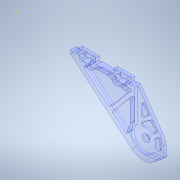
# Autodesk Inventor part: 後ろウィング固定フレームver2
Saved by Autodesk Inventor 2020.2 (Build 242310000, 310)
## iProperties
Created: 2020-05-07
Part Number: 後ろウィング固定フレームver2
Material: ポリカーボネート、クリア
Document SubType Name: Modeling
Designer: mozar
Density: 1.2 g/cm^3
Appearance: ポリカーボネート - クリア
Mass: 7.61117 g
Surface Area: 65.4566 cm^2
Volume: 6.34264 cm^3
Author: mozar
Autodesk Inventor part; units mm, degrees
(part 1 of 2)
ref_plane "YZ Plane" through (0, 0, 0) normal (1, 0, 0) x (0, 1, 0)
ref_plane "XZ Plane" through (0, 0, 0) normal (0, 1, 0) x (-1, 0, 0)
ref_plane "XY Plane" through (0, 0, 0) normal (0, 0, 1) x (1, 0, 0)
sketch "スケッチ1" plane through (0, 0, 0) normal (0, 0, 1) x (1, 0, 0)
  line L0 (-101.5, 48) -> (108.5, 48)
  circle A0 centre (111.885, -39) radius 4
  circle A1 centre (191.8767, -37.843) radius 4
  circle A2 centre (111.885, -39) radius 7
  circle A3 centre (191.8767, -37.843) radius 7
  line L1 (191.8767, -37.843) -> (111.885, -39) construction
  line L2 (191.7754, -30.8437) -> (111.7838, -32.0007)
  line L3 (111.9863, -45.9993) -> (191.9779, -44.8422)
  arc A4 (191.9779, -44.8422) -> (191.7754, -30.8437) centre (191.8767, -37.843) ccw
  arc A5 (111.7838, -32.0007) -> (111.9863, -45.9993) centre (111.885, -39) ccw
  line L4 (193.5423, -31.044) -> (241.7048, -42.843)
  circle A6 centre (234.5664, -71.9813) radius 30
  line L5 (262.5874, -82.6971) -> (213.7253, -50.4025)
  line L6 (213.7253, -50.4025) -> (190.2111, -44.6419)
  line L7 (264.5664, -121.5429) -> (264.5664, -63.2267)
  line L8 (111.885, -39) -> (111.885, 41) construction
  line L9 (118.885, -39) -> (118.885, 41)
  line L10 (104.885, 41) -> (104.885, -39)
  arc A7 (104.885, -39) -> (118.885, -39) centre (111.885, -39) ccw
  arc A8 (118.885, 41) -> (104.885, 41) centre (111.885, 41) ccw
  circle A9 centre (58.2383, 51.482) radius 30
  line L11 (113.5581, 34.2029) -> (65.4084, 22.3514)
  line L12 (28.4411, 48) -> (86.7041, 42.0109)
  line L13 (86.7041, 42.0109) -> (110.212, 47.7971)
  circle A10 centre (113.5, -20) radius 68
  line L14 (315.3272, -100.5855) -> (70.6004, 104.7647)
  line L15 (253.8501, -49) -> (111.885, -39)
  arc A11 (93.5924, -27.1048) -> (135.371, -5.9244) centre (95.0604, 21.7941) ccw
  arc A12 (135.371, -5.9244) -> (135.8476, -3.6716) centre (132.899, -4.2246) ccw
  arc A13 (135.8476, -3.6716) -> (83.1833, 18.5565) centre (102.1579, -9.9896) ccw
  line L16 (111.885, -39) -> (112.7472, 40.9954) construction
  line L17 (118.8846, -39.0754) -> (119.7468, 40.9199)
  line L18 (105.7476, 41.0708) -> (104.8855, -38.9246)
  arc A14 (104.8855, -38.9246) -> (118.8846, -39.0754) centre (111.885, -39) ccw
  arc A15 (119.7468, 40.9199) -> (105.7476, 41.0708) centre (112.7472, 40.9954) ccw
  line L19 (164.9949, 48) -> (164.9949, 26)
  line L20 (164.9949, 26) -> (327.4949, -102)
  circle A16 centre (116.2926, -40) radius 68
  circle A17 centre (-98.885, 0) radius 67.5
  line L21 (321.3633, -8.501) -> (-152.6681, 78.4982)
  line L22 (104.8897, -3) -> (104.8897, 0)
  line L23 (104.8897, -3) -> (64.4443, -3)
  line L24 (72.0656, 0) -> (104.8897, 0)
  circle A18 centre (83.3769, -17.5) radius 13.85
  line L25 (198.5102, -35.6076) -> (190.7791, -12.6656)
  line L26 (185.2432, -40.0784) -> (169.4082, 6.912)
  circle A19 centre (197.8374, 16.4922) radius 30
  line L27 (190.7791, -12.6656) -> (191.8767, 45.8941)
  circle A20 centre (191.8767, -37.843) radius 83.7371
  line L28 (191.8767, 45.8941) -> (191.8767, -37.843)
  line L29 (96.8897, -3) -> (96.8897, -6)
  line L30 (96.8897, -6) -> (87.8897, -6)
  line L31 (87.8897, -6) -> (87.8897, -3)
  line L32 (76.4443, -3) -> (76.4443, -6)
  line L33 (76.4443, -6) -> (67.4443, -6)
  line L34 (67.4443, -6) -> (67.4443, -3)
  line L35 (99.8897, -3) -> (99.8897, 0)
  line L36 (99.8897, 0) -> (84.8897, 0)
  line L37 (84.8897, 0) -> (84.8897, -3)
  line L38 (79.4443, -3) -> (79.4443, 0)
  line L39 (79.4443, 0) -> (64.4443, 0)
  line L40 (64.4443, 0) -> (64.4443, -3)
  line L41 (64.4443, 0) -> (59.4443, 0)
  line L42 (59.4443, 0) -> (59.4443, -3)
  line L43 (59.4443, -3) -> (64.4443, -3)
  line L44 (59.4443, -3) -> (59.4443, -6)
  circle A21 centre (111.885, -39) radius 1.5
  circle A22 centre (111.885, -39) radius 9
  circle A23 centre (111.885, -39) radius 10
  circle A24 centre (111.885, -39) radius 15
  line L45 (121.0577, -50.8686) -> (142.9273, -50.5523)
  line L46 (121.0577, -50.8686) -> (127.6513, -45.7727)
  line L47 (127.6513, -45.7727) -> (126.8081, -37.4821)
  line L48 (124.1514, -30.3665) -> (104.8897, -3)
  line L49 (101.0602, -49.3838) -> (59.4443, -6)
  circle A25 centre (95.8897, -6) radius 1
  circle A26 centre (88.8897, -6) radius 1
  circle A27 centre (95.8897, -3) radius 1
  circle A28 centre (88.8897, -3) radius 1
  circle A29 centre (100.8897, -3) radius 1
  circle A30 centre (83.8897, -3) radius 1
  circle A31 centre (80.4443, -3) radius 1
  circle A32 centre (75.4443, -6) radius 1
  circle A33 centre (68.4443, -6) radius 1
  circle A34 centre (75.4443, -3) radius 1
  circle A35 centre (68.4443, -3) radius 1
  circle A36 centre (63.4443, -3) radius 1
  point P0 (0, 0)
  point P1 (151.8809, -38.4215)
  point P2 (111.885, 1)
  point P3 (105.885, 0)
  point P4 (105.885, 0)
  point P5 (23.7328, -42.729)
  point P6 (112.3161, 0.9977)
  point P7 (99.8897, -1.5)
  point P8 (76.4443, -4.5)
  point P9 (74.4443, -6)
  point P10 (69.4443, -6)
  point P11 (69.4443, -3)
  point P12 (74.4443, -3)
  point P13 (82.8897, -3)
  point P14 (81.4443, -3)
  point P15 (62.4443, -3)
  point P16 (101.8897, -3)
  point P17 (89.8897, -3)
  point P18 (94.8897, -3)
  point P19 (94.8897, -6)
  point P20 (89.8897, -6)
  point P21 (118.9616, -31.9344)
  point P22 (118.9245, -31.8974)
  point P23 (118.962, -31.8969)
  point P24 (119.127, -45.896)
  point P25 (104.885, -3)
  point P26 (104.885, -31.8586)
  dimension "d27" = 167.4741
  dimension "d0" = 8
  dimension "d1" = 8
  dimension "d2" = 3
  dimension "d3" = 3
  dimension "d4" = 80
  dimension "d5" = 14
  dimension "d6" = 14
  dimension "d7" = 60
  dimension "d8" = 14
  dimension "d9" = 60
  dimension "d10" = 14
  dimension "d11" = 6
  dimension "d12" = 40
  dimension "d13" = 13.271
  dimension "d14" = 14
  dimension "d15" = 10
  dimension "d16" = 5
  dimension "d17" = 22
  dimension "d18" = 150
  dimension "d19" = 162.5
  dimension "d20" = 0
  dimension "d21" = 136
  dimension "d22" = 136
  dimension "d23" = 135
  dimension "d24" = 38.227
  dimension "d25" = 25
  dimension "d26" = 60
  dimension "d28" = 5
  dimension "d29" = 3
  dimension "d30" = 5
  dimension "d31" = 3
  dimension "d32" = 3
  dimension "d33" = 5
  dimension "d34" = 1
  dimension "d35" = 5
  dimension "d36" = 5
  dimension "d37" = 2
  dimension "d38" = 2
  dimension "d39" = 2
  dimension "d40" = 2
  dimension "d41" = 2
  dimension "d42" = 2
  dimension "d43" = 2
  dimension "d44" = 2
  dimension "d45" = 2
  dimension "d46" = 2
  dimension "d47" = 2
  dimension "d48" = 2
  constraints: 104 end point, 46 tangent, 37 point on circle, 36 centre point, 14 vertical, 8 point on line, 7 equal length, 7 horizontal, 5 coincident, 5 midpoint, 5 parallel, 1 concentric, 1 perpendicular, 1 vertical alignment, 25 other
  measures "d0" diameter of A0
  measures "d1" diameter of A1
  measures "d2" radial gap between concentric circles of A0 A2
  measures "d3" radial gap between concentric circles of A1 A3
  measures "d4" distance of L1.start L1.end
  measures "d5" diameter of A5
  measures "d6" distance from line of L4 L5.end
  measures "d7" diameter of A6
  measures "d8" diameter of A8
  measures "d9" diameter of A9
  measures "d10" distance from line of L11 L12.end
  measures "d11" horizontal distance of L1.end point (105.885, 0)
  measures "d12" angle of L14 L0
  measures "d14" diameter of A15
  measures "d15" vertical distance of L15.start L1.end
  measures "d16" vertical distance of L1.start L4.end
  measures "d17" distance of L19.start L19.end
  measures "d18" vertical distance of L19.start L20.end
  measures "d19" distance from line of L19 L20.end
  measures "d20" distance from line of L19.start L0
  measures "d21" diameter of A10
  measures "d22" diameter of A16
  measures "d23" diameter of A17
  measures "d24" angle of L0 L20
  measures "d25" distance from line of L5.start L20
  measures "d26" diameter of A19
  measures "d28" distance between parallel lines of L35 L22
  measures "d29" distance of L41.end L42.end
  measures "d30" distance of L42.end L40.end
  measures "d31" distance of L42.end L44.end
  measures "d32" diameter of A21
  measures "d33" radial gap between concentric circles of A0 A22
  measures "d34" radial gap between concentric circles of A22 A23
  measures "d35" radial gap between concentric circles of A23 A24
  measures "d36" distance between parallel lines of L3 L45
  measures "d37" diameter of A25
  measures "d38" diameter of A26
  measures "d39" diameter of A27
  measures "d40" diameter of A28
  measures "d41" diameter of A29
  measures "d42" diameter of A30
  measures "d43" diameter of A31
  measures "d44" diameter of A32
  measures "d45" diameter of A33
  measures "d46" diameter of A34
  measures "d47" diameter of A35
  measures "d48" diameter of A36
extrude "押し出し1" add sketch "スケッチ1" against normal blind 5 contours A24 A11 L10 A23 A20 | A20 A23 L3 A24 | L43 A36 L23 L34 A33 L33 A32 A18 L49 L44 | L46 A24 L3 | L3 A24 L15 L47 | A23 L10 A22 A20 | A20 A22 L3 A23 | L49 A18 L30 A25 L29 L23 A29 L10 A24 | L39 L24 L38 L23 A34 A35 L40 | L3 A23 L15 A24 | L15 A24 L47 | A22 L10 A2 A20 | A20 A2 L3 A22 | A23 L18 A22 L10 | L10 A11 L18 A23 | L3 A22 L15 A23 | A24 L10 A11 | L49 A18 A32 L32 A31 A30 L31 A26 L30 | L15 A23 L17 L2 A24 | L2 L17 A24 | A20 A0 L15 A2 | A2 A20 A0 | A22 L18 L10 | L3 A2 L15 A22 | L10 A24 L18 A11 | A23 A20 A22 L18 | L18 A11 A20 A23 | L15 A22 L17 A23 | L10 L23 L48 L18 A24 | L35 L23 A27 A28 L37 L24 | L48 A20 A24 L18 | L17 A23 L2 | L2 A23 L9 A24 L17 | A24 L17 L48 | A20 A0 | A0 A20 | L18 A22 A20 A2 | L15 A2 L17 A22 | L18 A24 A20 A11 | A23 L9 L2 A22 A20 | A20 A11 A24 L9 A23 | A31 A18 L32 L23 | L48 A11 A24 A20 | A23 L17 A22 L9 L2 | L2 L9 A23 | A24 L9 L48 L17 | L15 A0 A20 A2 | A20 A22 L2 A2 | A20 A24 A11 | A18 A30 L23 L31 | L23 A30 A18 A31 | L48 L9 A24 A11 | L9 A22 L2 | L17 L9 A22 | L2 A22 L9 A2
extrude "押し出し2" cut sketch "スケッチ1" against normal blind 2.55 contours L3 A24 L15 L47 | A23 L10 A22 A20 | A20 A22 L3 A23 | L3 A23 L15 A24 | L15 A24 L47 | A22 L10 A2 A20 | A20 A2 L3 A22 | A23 L18 A22 L10 | L10 A11 L18 A23 | L3 A22 L15 A23 | L15 A23 L17 L2 A24 | L2 L17 A24 | A20 A0 L15 A2 | A2 A20 A0 | A22 L18 L10 | L3 A2 L15 A22 | L10 A24 L18 A11 | A23 A20 A22 L18 | L18 A11 A20 A23 | L15 A22 L17 A23 | L10 L23 L48 L18 A24 | L48 A20 A24 L18 | L17 A23 L2 | L2 A23 L9 A24 L17 | A24 L17 L48 | A20 A0 | A0 A20 | L18 A22 A20 A2 | L15 A2 L17 A22 | L18 A24 A20 A11 | A23 L9 L2 A22 A20 | A20 A11 A24 L9 A23 | L48 A11 A24 A20 | A23 L17 A22 L9 L2 | L2 L9 A23 | A24 L9 L48 L17 | L15 A0 A20 A2 | A20 A22 L2 A2 | A20 A24 A11 | L48 L9 A24 A11 | L9 A22 L2 | L17 L9 A22 | L2 A22 L9 A2 | A21
sketch "スケッチ2" plane through (0, 0, 0) normal (0, 0, 1) x (1, 0, 0)
  line L0 (87.8897, -6) -> (87.8897, -3) projected
  arc A0 (89.8897, -3) -> (87.8897, -3) centre (88.8897, -3) ccw projected
  line L1 (89.8897, -3) -> (94.8897, -3) projected
  arc A1 (96.8897, -3) -> (94.8897, -3) centre (95.8897, -3) ccw projected
  line L2 (96.8897, -3) -> (96.8897, -6) projected
  arc A2 (94.8897, -6) -> (96.8897, -6) centre (95.8897, -6) ccw projected
  line L3 (94.8897, -6) -> (89.8897, -6) projected
  arc A3 (87.8897, -6) -> (89.8897, -6) centre (88.8897, -6) ccw projected
  arc A4 (67.4443, -6) -> (69.4443, -6) centre (68.4443, -6) ccw projected
  line L4 (67.4443, -6) -> (67.4443, -3) projected
  arc A5 (69.4443, -3) -> (67.4443, -3) centre (68.4443, -3) ccw projected
  line L5 (69.4443, -3) -> (74.4443, -3) projected
  arc A6 (76.4443, -3) -> (74.4443, -3) centre (75.4443, -3) ccw projected
  line L6 (76.4443, -3) -> (76.4443, -6) projected
  arc A7 (74.4443, -6) -> (76.4443, -6) centre (75.4443, -6) ccw projected
  line L7 (74.4443, -6) -> (69.4443, -6) projected
  line L8 (127.6513, -45.7727) -> (119.127, -45.896) projected
  arc A8 (104.885, -31.8586) -> (119.127, -45.896) centre (111.885, -39) ccw projected
  line L9 (104.885, -31.8586) -> (104.885, -3) projected
  line L10 (104.885, -3) -> (101.8897, -3) projected
  arc A9 (99.8897, -3) -> (101.8897, -3) centre (100.8897, -3) ccw projected
  line L11 (99.8897, -3) -> (99.8897, 0) projected
  line L12 (99.8897, 0) -> (84.8897, 0) projected
  line L13 (84.8897, 0) -> (84.8897, -3) projected
  arc A10 (82.8897, -3) -> (84.8897, -3) centre (83.8897, -3) ccw projected
  line L14 (82.8897, -3) -> (81.4443, -3) projected
  arc A11 (79.4443, -3) -> (81.4443, -3) centre (80.4443, -3) ccw projected
  line L15 (79.4443, -3) -> (79.4443, 0) projected
  line L16 (79.4443, 0) -> (64.4443, 0) projected
  line L17 (64.4443, 0) -> (64.4443, -3) projected
  arc A12 (62.4443, -3) -> (64.4443, -3) centre (63.4443, -3) ccw projected
  line L18 (62.4443, -3) -> (59.4443, -3) projected
  line L19 (59.4443, -3) -> (59.4443, -6) projected
  line L20 (59.4443, -6) -> (101.0602, -49.3838) projected
  arc A13 (101.0602, -49.3838) -> (121.0577, -50.8686) centre (111.885, -39) ccw projected
  line L21 (121.0577, -50.8686) -> (127.6513, -45.7727) projected
  circle A14 centre (111.885, -39) radius 1.5 projected
  circle A15 centre (111.885, -39) radius 3
  point P0 (0, 0)
  dimension "d53" = 6
  constraints: 1 centre point, 1 coincident
  measures "d53" diameter of A15
extrude "押し出し3" cut sketch "スケッチ2" against normal blind 3 contours A15
sketch "スケッチ3" plane through (0, 0, 0) normal (0, 0, 1) x (1, 0, 0)
  line L0 (87.8897, -6) -> (87.8897, -3) projected
  arc A0 (89.8897, -3) -> (87.8897, -3) centre (88.8897, -3) ccw projected
  line L1 (89.8897, -3) -> (94.8897, -3) projected
  arc A1 (96.8897, -3) -> (94.8897, -3) centre (95.8897, -3) ccw projected
  line L2 (96.8897, -3) -> (96.8897, -6) projected
  arc A2 (94.8897, -6) -> (96.8897, -6) centre (95.8897, -6) ccw projected
  line L3 (94.8897, -6) -> (89.8897, -6) projected
  arc A3 (87.8897, -6) -> (89.8897, -6) centre (88.8897, -6) ccw projected
  arc A4 (67.4443, -6) -> (69.4443, -6) centre (68.4443, -6) ccw projected
  line L4 (67.4443, -6) -> (67.4443, -3) projected
  arc A5 (69.4443, -3) -> (67.4443, -3) centre (68.4443, -3) ccw projected
  line L5 (69.4443, -3) -> (74.4443, -3) projected
  arc A6 (76.4443, -3) -> (74.4443, -3) centre (75.4443, -3) ccw projected
  line L6 (76.4443, -3) -> (76.4443, -6) projected
  arc A7 (74.4443, -6) -> (76.4443, -6) centre (75.4443, -6) ccw projected
  line L7 (74.4443, -6) -> (69.4443, -6) projected
  line L8 (127.6513, -45.7727) -> (119.127, -45.896) projected
  arc A8 (104.885, -31.8586) -> (119.127, -45.896) centre (111.885, -39) ccw projected
  line L9 (104.885, -31.8586) -> (104.885, -3) projected
  line L10 (104.885, -3) -> (101.8897, -3) projected
  arc A9 (99.8897, -3) -> (101.8897, -3) centre (100.8897, -3) ccw projected
  line L11 (99.8897, -3) -> (99.8897, 0) projected
  line L12 (99.8897, 0) -> (84.8897, 0) projected
  line L13 (84.8897, 0) -> (84.8897, -3) projected
  arc A10 (82.8897, -3) -> (84.8897, -3) centre (83.8897, -3) ccw projected
  line L14 (82.8897, -3) -> (81.4443, -3) projected
  arc A11 (79.4443, -3) -> (81.4443, -3) centre (80.4443, -3) ccw projected
  line L15 (79.4443, -3) -> (79.4443, 0) projected
  line L16 (79.4443, 0) -> (64.4443, 0) projected
  line L17 (64.4443, 0) -> (64.4443, -3) projected
  arc A12 (62.4443, -3) -> (64.4443, -3) centre (63.4443, -3) ccw projected
  line L18 (62.4443, -3) -> (59.4443, -3) projected
  line L19 (59.4443, -3) -> (59.4443, -6) projected
  line L20 (59.4443, -6) -> (101.0602, -49.3838) projected
  arc A13 (101.0602, -49.3838) -> (121.0577, -50.8686) centre (111.885, -39) ccw projected
  line L21 (121.0577, -50.8686) -> (127.6513, -45.7727) projected
  line L22 (99.8897, 0) -> (99.8897, -3) projected
  line L23 (99.8897, 0) -> (64.4443, 0)
  line L24 (64.4443, 0) -> (64.4443, -3)
  line L25 (64.4443, -3) -> (99.8897, -3)
  line L26 (99.8897, -3) -> (99.8897, 0)
  point P0 (0, 0)
  constraints: 8 end point, 2 parallel, 1 horizontal, 1 perpendicular
extrude "押し出し4" cut sketch "スケッチ3" against normal blind 2 contours L25 L13 L12 L11 A1 L1 A0 | A0 L25 | L25 L14 L15 L23 L13 | A1 L25 | L15 L25 A6 L5 A5 L17 L16 | L25 A6 | A5 L25
sketch "スケッチ4" plane through (0, 0, -5) normal (0, 0, -1) x (-1, 0, 0)
  circle A0 centre (-111.885, -39) radius 3 projected
  line L0 (-104.885, -3) -> (-104.8897, -3) projected
  line L1 (-104.885, -31.8586) -> (-104.885, -3) projected
  arc A1 (-119.127, -45.896) -> (-104.885, -31.8586) centre (-111.885, -39) ccw projected
  line L2 (-127.6513, -45.7727) -> (-119.127, -45.896) projected
  line L3 (-126.8081, -37.4821) -> (-127.6513, -45.7727) projected
  arc A2 (-124.1514, -30.3665) -> (-126.8081, -37.4821) centre (-111.885, -39) ccw projected
  line L4 (-104.8897, -3) -> (-124.1514, -30.3665) projected
  circle A3 centre (-111.885, -39) radius 1.5 projected
  point P0 (0, 0)
sketch "スケッチ6" plane through (0, 0, -5) normal (0, 0, -1) x (-1, 0, 0)
  line L0 (-79.4443, 0) -> (-79.4443, -3) projected
  line L1 (-64.4443, 0) -> (-79.4443, 0) projected
  line L2 (-64.4443, -3) -> (-64.4443, 0) projected
  line L3 (-67.4443, -3) -> (-64.4443, -3) projected
  arc A0 (-67.4443, -3) -> (-69.4443, -3) centre (-68.4443, -3) ccw projected
  line L4 (-74.4443, -3) -> (-69.4443, -3) projected
  arc A1 (-74.4443, -3) -> (-76.4443, -3) centre (-75.4443, -3) ccw projected
  line L5 (-79.4443, -3) -> (-76.4443, -3) projected
  arc A2 (-94.8897, -3) -> (-96.8897, -3) centre (-95.8897, -3) ccw projected
  line L6 (-99.8897, -3) -> (-96.8897, -3) projected
  line L7 (-99.8897, 0) -> (-99.8897, -3) projected
  line L8 (-84.8897, 0) -> (-99.8897, 0) projected
  line L9 (-84.8897, -3) -> (-84.8897, 0) projected
  line L10 (-87.8897, -3) -> (-84.8897, -3) projected
  arc A3 (-87.8897, -3) -> (-89.8897, -3) centre (-88.8897, -3) ccw projected
  line L11 (-94.8897, -3) -> (-89.8897, -3) projected
  point P0 (0, 0)
sketch "スケッチ8" plane through (0, 0, -5) normal (0, 0, -1) x (-1, 0, 0)
  line L0 (-84.8897, -3) -> (-87.8897, -3)
  line L1 (-87.8897, -3) -> (-87.8897, -6)
  arc A0 (-89.8897, -6) -> (-87.8897, -6) centre (-88.8897, -6) ccw
  line L2 (-89.8897, -6) -> (-94.8897, -6)
  arc A1 (-96.8897, -6) -> (-94.8897, -6) centre (-95.8897, -6) ccw
  line L3 (-96.8897, -6) -> (-96.8897, -3)
  line L4 (-96.8897, -3) -> (-99.8897, -3)
  arc A2 (-101.8897, -3) -> (-99.8897, -3) centre (-100.8897, -3) ccw
  line L5 (-101.8897, -3) -> (-104.885, -3)
  line L6 (-104.885, -3) -> (-104.885, -31.8586)
  arc A3 (-119.127, -45.896) -> (-104.885, -31.8586) centre (-111.885, -39) ccw
  line L7 (-119.127, -45.896) -> (-127.6513, -45.7727)
  line L8 (-127.6513, -45.7727) -> (-121.0577, -50.8686)
  arc A4 (-121.0577, -50.8686) -> (-101.0602, -49.3838) centre (-111.885, -39) ccw
  line L9 (-101.0602, -49.3838) -> (-59.4443, -6)
  line L10 (-59.4443, -6) -> (-59.4443, -3)
  line L11 (-59.4443, -3) -> (-62.4443, -3)
  arc A5 (-64.4443, -3) -> (-62.4443, -3) centre (-63.4443, -3) ccw
  line L12 (-64.4443, -3) -> (-67.4443, -3)
  line L13 (-67.4443, -3) -> (-67.4443, -6)
  arc A6 (-69.4443, -6) -> (-67.4443, -6) centre (-68.4443, -6) ccw
  line L14 (-69.4443, -6) -> (-74.4443, -6)
  arc A7 (-76.4443, -6) -> (-74.4443, -6) centre (-75.4443, -6) ccw
  line L15 (-76.4443, -6) -> (-76.4443, -3)
  line L16 (-76.4443, -3) -> (-79.4443, -3)
  arc A8 (-81.4443, -3) -> (-79.4443, -3) centre (-80.4443, -3) ccw
  line L17 (-81.4443, -3) -> (-82.8897, -3)
  arc A9 (-84.8897, -3) -> (-82.8897, -3) centre (-83.8897, -3) ccw
  line L18 (-66.4443, -6) -> (-57.4443, -6)
  line L19 (-57.4443, -6) -> (-57.4443, -3)
  line L20 (-57.4443, -3) -> (-66.4443, -3)
  line L21 (-66.4443, -3) -> (-66.4443, -6)
  line L22 (-69.4443, -6) -> (-74.4443, -6)
  line L23 (-64.4443, -3) -> (-67.4443, -3)
  circle A10 centre (-65.4443, -3) radius 1
  circle A11 centre (-65.4443, -6) radius 1
  circle A12 centre (-58.4443, -3) radius 1
  circle A13 centre (-58.4443, -6) radius 1
  line L24 (-54.4443, 0) -> (-54.4443, -6)
  line L25 (-61.0901, -9) -> (-62.7986, -9)
  line L26 (-69.4443, -6) -> (-69.4443, 0)
  line L27 (-69.4443, 0) -> (-54.4443, 0)
  circle A14 centre (-65.4443, -6) radius 4
  circle A15 centre (-58.4443, -6) radius 4
  line L28 (-64.4443, 0) -> (-64.4443, -3)
  line L29 (-79.4443, -3) -> (-79.4443, 0)
  line L30 (-69.4443, 0) -> (-54.4443, 0)
  line L31 (-54.4443, 0) -> (-54.4443, -3)
  line L32 (-54.4443, -3) -> (-69.4443, -3)
  line L33 (-69.4443, -3) -> (-69.4443, 0)
  line L34 (-54.4443, -3) -> (-49.4443, -3)
  line L35 (-49.4443, -3) -> (-49.4443, -6)
  line L36 (-49.4443, -6) -> (-54.4443, -6)
  line L37 (-54.4443, -6) -> (-54.4443, -3)
  circle A16 centre (-53.4443, -3) radius 1
  circle A17 centre (-70.4443, -3) radius 1
  line L38 (-76.4443, -3) -> (-69.4443, -3)
  line L39 (-79.4443, 0) -> (-64.4443, 0)
  line L40 (-79.4443, 0) -> (-64.4443, 0)
  line L41 (-81.4443, -3) -> (-79.4443, -3)
  point P0 (0, 0)
  point P1 (0, 0)
  point P2 (-61.9443, -3)
  point P3 (-52.4443, -3)
  point P4 (-71.4443, -3)
  point P5 (-59.4443, -6)
  point P6 (-64.4443, -6)
  point P7 (-68.0901, -3)
  point P8 (-64.4443, -2.127)
  point P9 (-62.4911, -3.3022)
  point P10 (-61.0901, -3)
  point P11 (-61.9443, -4.0635)
  point P12 (-61.9443, -7.9365)
  point P13 (-52.4443, -3)
  point P14 (-59.4443, -6)
  point P15 (-64.4443, -6)
  point P16 (-71.4443, -3)
  dimension "d68" = 9
  dimension "d69" = 3
  dimension "d70" = 10
  dimension "d71" = 2
  dimension "d72" = 2
  dimension "d73" = 2
  dimension "d74" = 2
  dimension "d75" = 3
  dimension "d76" = 3
  dimension "d77" = 3
  dimension "d78" = 3
  dimension "d79" = 15
  dimension "d80" = 15
  dimension "d81" = 3
  dimension "d82" = 3
  dimension "d83" = 15
  dimension "d84" = 3
  dimension "d85" = 10
  dimension "d86" = 2
  dimension "d87" = 2
  constraints: 84 end point, 24 point on circle, 18 centre point, 8 parallel, 7 point on line, 7 tangent, 4 horizontal, 4 perpendicular, 2 midpoint, 1 collinear
  measures "d68" distance of L20.end L19.end
  measures "d69" distance of L19.end L18.end
  measures "d70" distance between parallel lines of L15 L21
  measures "d71" diameter of A10
  measures "d72" diameter of A11
  measures "d73" diameter of A12
  measures "d74" diameter of A13
  measures "d75" distance between parallel lines of L19 L24
  measures "d76" radial gap between concentric circles of A11 A14
  measures "d77" radial gap between concentric circles of A13 A15
  measures "d78" distance between parallel lines of L14 L25
  measures "d79" distance between parallel lines of L28 L29
  measures "d80" distance of L31.end L32.end
  measures "d81" distance of L30.end L31.end
  measures "d82" distance between parallel lines of L32 L27
  measures "d83" distance between parallel lines of L31 L33
  measures "d84" distance of L34.end L35.end
  measures "d85" distance between parallel lines of L35 L10
  measures "d86" diameter of A16
  measures "d87" diameter of A17
extrude "押し出し10" cut sketch "スケッチ8" against normal blind 10 contours L29 L39 L26 A17 L38 L16 | A17 L38 | L27 L28 A14 L32 L26 picked at (-70.1948, -2.6194)
extrude "押し出し11" add sketch "スケッチ8" against normal blind 5 contours L41 A8 | L38 A17 L26 L14 A7 L15 | L38 A17 | L32 A14 L26 | A14 L32 L13 A6 picked at (-70.6938, -3.3806)
extrude "押し出し12" cut sketch "スケッチ8" against normal blind 10 contours A14 A10 L12 L32 | L28 A10 A14 | A10 L12 | A10 L12
extrude "押し出し13" add sketch "スケッチ8" against normal blind 5 contours L27 L28 A14 L32 L26 | L27 L24 L32 A15 L11 L20 A14 L28 | A14 L32 L13 A6 | A6 L13 L12 L21 A11 L18 A15 A14 | A14 A10 L12 L32 | L28 A10 A14 | A14 L20 L28 | A10 L12 | A16 L34 L35 L36 L24 | L24 A15 L32 | A14 A5 L20 | L20 A5 A14 | A10 L12 | A5 A14 A15 L18 A11 L21 A10 | A15 L18 A14 | A14 L18 L9 A15 | A15 L9 A13 L19 L32 | L32 A12 A15 | A14 A15 L11 L10 L18 | L18 A15 A14 | A11 L18 | L18 A11 | A12 L20 | A12 L11 A15 | A12 L20 | L19 A13 L10 A12 | A13 L18 | L18 A13
extrude "押し出し14" cut sketch "スケッチ8" against normal blind 10 contours L38 A17 | A10 L12 | A14 A5 L20 | L20 A5 A14 | A10 L12 | A5 A14 A15 L18 A11 L21 A10 | L11 A15 A14 A5 | A14 A15 L11 L10 L18 | L18 A15 A14 | A11 L18 | L18 A11 | A12 L20 | A12 L20 | L19 A13 L10 A12 | A13 L18 | L18 A13 picked at (-70.6938, -3.3806) picked at (-61.7965, -5.7765)
sketch "スケッチ9" plane through (0, 0, 0) normal (0, 0, 1) x (1, 0, 0)
  arc A0 (69.4443, -3) -> (71.4443, -3) centre (70.4443, -3) ccw projected
  line L0 (69.4443, -3) -> (69.4443, 0) projected
  line L1 (69.4443, 0) -> (54.4443, 0) projected
  line L2 (54.4443, 0) -> (54.4443, -3) projected
  arc A1 (52.4443, -3) -> (54.4443, -3) centre (53.4443, -3) ccw projected
  line L3 (52.4443, -3) -> (49.4443, -3) projected
  line L4 (49.4443, -3) -> (49.4443, -6) projected
  line L5 (49.4443, -6) -> (54.4443, -6) projected
  arc A2 (54.4443, -6) -> (61.6887, -8.3397) centre (58.4443, -6) ccw projected
  line L6 (61.6887, -8.3397) -> (101.0602, -49.3838) projected
  arc A3 (101.0602, -49.3838) -> (121.0577, -50.8686) centre (111.885, -39) ccw projected
  line L7 (121.0577, -50.8686) -> (127.6513, -45.7727) projected
  line L8 (127.6513, -45.7727) -> (119.127, -45.896) projected
  arc A4 (104.885, -31.8586) -> (119.127, -45.896) centre (111.885, -39) ccw projected
  line L9 (104.885, -31.8586) -> (104.885, -3) projected
  line L10 (104.885, -3) -> (101.8897, -3) projected
  arc A5 (99.8897, -3) -> (101.8897, -3) centre (100.8897, -3) ccw projected
  line L11 (99.8897, -3) -> (96.8897, -3) projected
  line L12 (96.8897, -3) -> (96.8897, -6) projected
  arc A6 (94.8897, -6) -> (96.8897, -6) centre (95.8897, -6) ccw projected
  line L13 (94.8897, -6) -> (89.8897, -6) projected
  arc A7 (87.8897, -6) -> (89.8897, -6) centre (88.8897, -6) ccw projected
  line L14 (87.8897, -6) -> (87.8897, -3) projected
  line L15 (87.8897, -3) -> (84.8897, -3) projected
  arc A8 (82.8897, -3) -> (84.8897, -3) centre (83.8897, -3) ccw projected
  line L16 (82.8897, -3) -> (71.4443, -3) projected
  arc A9 (66.4443, -3) -> (64.4443, -3) centre (65.4443, -3) ccw projected
  line L17 (66.4443, -3) -> (66.4443, -6) projected
  arc A10 (64.4443, -6) -> (66.4443, -6) centre (65.4443, -6) ccw projected
  line L18 (64.4443, -6) -> (59.4443, -6) projected
  arc A11 (57.4443, -6) -> (59.4443, -6) centre (58.4443, -6) ccw projected
  line L19 (57.4443, -6) -> (57.4443, -3) projected
  arc A12 (59.4443, -3) -> (57.4443, -3) centre (58.4443, -3) ccw projected
  line L20 (59.4443, -3) -> (64.4443, -3) projected
  line L21 (69.4443, 0) -> (69.4443, -3) projected
  line L22 (69.4443, -3) -> (54.4443, -3)
  circle A13 centre (111.885, -39) radius 1.5 projected
  arc A14 (101.0602, -49.3838) -> (121.0577, -50.8686) centre (111.885, -39) ccw projected
  circle A15 centre (111.885, -39) radius 15
  line L23 (49.4443, -6) -> (49.4443, -3) projected
  line L24 (102.2194, -50.4706) -> (49.4443, -6)
  point P0 (0, 0)
  constraints: 4 end point, 2 point on circle, 1 centre point, 1 coincident, 1 perpendicular, 1 tangent
extrude "押し出し15" add sketch "スケッチ9" against normal blind 5 contours L5 A2 L6 A3 L24
extrude "押し出し16" cut sketch "スケッチ9" against normal blind 2 contours L22 A9 L20 A12 L2 L1 L0
sketch "スケッチ10" plane through (0, 0, 0) normal (0, 0, 1) x (1, 0, 0)
  line L0 (57.4443, -3) -> (54.4443, -3) projected
  arc A0 (52.4443, -3) -> (54.4443, -3) centre (53.4443, -3) ccw projected
  line L1 (52.4443, -3) -> (49.4443, -3) projected
  line L2 (49.4443, -3) -> (49.4443, -6) projected
  line L3 (49.4443, -6) -> (102.2194, -50.4706) projected
  arc A1 (102.2194, -50.4706) -> (121.0577, -50.8686) centre (111.885, -39) ccw projected
  line L4 (121.0577, -50.8686) -> (127.6513, -45.7727) projected
  line L5 (127.6513, -45.7727) -> (119.127, -45.896) projected
  arc A2 (104.885, -31.8586) -> (119.127, -45.896) centre (111.885, -39) ccw projected
  line L6 (104.885, -31.8586) -> (104.885, -3) projected
  line L7 (104.885, -3) -> (101.8897, -3) projected
  arc A3 (99.8897, -3) -> (101.8897, -3) centre (100.8897, -3) ccw projected
  line L8 (99.8897, -3) -> (96.8897, -3) projected
  line L9 (96.8897, -3) -> (96.8897, -6) projected
  arc A4 (94.8897, -6) -> (96.8897, -6) centre (95.8897, -6) ccw projected
  line L10 (94.8897, -6) -> (89.8897, -6) projected
  arc A5 (87.8897, -6) -> (89.8897, -6) centre (88.8897, -6) ccw projected
  line L11 (87.8897, -6) -> (87.8897, -3) projected
  line L12 (87.8897, -3) -> (84.8897, -3) projected
  arc A6 (82.8897, -3) -> (84.8897, -3) centre (83.8897, -3) ccw projected
  line L13 (82.8897, -3) -> (71.4443, -3) projected
  arc A7 (69.4443, -3) -> (71.4443, -3) centre (70.4443, -3) ccw projected
  line L14 (69.4443, -3) -> (66.4443, -3) projected
  line L15 (66.4443, -3) -> (66.4443, -6) projected
  arc A8 (64.4443, -6) -> (66.4443, -6) centre (65.4443, -6) ccw projected
  line L16 (64.4443, -6) -> (59.4443, -6) projected
  arc A9 (57.4443, -6) -> (59.4443, -6) centre (58.4443, -6) ccw projected
  line L17 (57.4443, -6) -> (57.4443, -3) projected
  circle A10 centre (111.885, -39) radius 3 projected
  line L18 (104.885, -3) -> (104.8897, -3) projected
  line L19 (104.885, -31.8586) -> (104.885, -3) projected
  arc A11 (104.885, -31.8586) -> (119.127, -45.896) centre (111.885, -39) ccw projected
  line L20 (127.6513, -45.7727) -> (119.127, -45.896) projected
  line L21 (126.8081, -37.4821) -> (127.6513, -45.7727) projected
  arc A12 (126.8081, -37.4821) -> (124.1514, -30.3665) centre (111.885, -39) ccw projected
  line L22 (104.8897, -3) -> (124.1514, -30.3665) projected
  line L23 (106.0857, -45.8824) -> (66.885, -12.8501)
  arc A13 (66.885, -12.8501) -> (72.4443, -6) centre (65.4443, -6) ccw
  line L24 (72.4443, -6) -> (72.4443, 3.7082)
  arc A14 (72.4443, 3.7082) -> (74.0499, -9) centre (70.4443, -3) ccw
  line L25 (74.0499, -9) -> (80.2841, -9)
  arc A15 (80.2841, -9) -> (81.8897, 3.7082) centre (83.8897, -3) ccw
  line L26 (81.8897, 3.7082) -> (81.8897, -6)
  arc A16 (81.8897, -6) -> (92.4952, -12) centre (88.8897, -6) ccw
  line L27 (92.4952, -12) -> (92.2841, -12)
  arc A17 (92.2841, -12) -> (98.885, -12.3268) centre (95.8897, -6) ccw
  line L28 (98.885, -12.3268) -> (98.885, -29.6726)
  arc A18 (98.885, -29.6726) -> (127.8557, -38.0317) centre (111.885, -39) ccw
  line L29 (127.8557, -38.0317) -> (117.3886, -46.1211)
  arc A19 (106.0857, -45.8824) -> (117.3886, -46.1211) centre (111.885, -39) ccw
  point P0 (0, 0)
  point P1 (83.1155, -9.9571)
  point P2 (71.2186, -9.9571)
  point P3 (95.9695, -37.3581)
  point P4 (92.3897, -12.0622)
  dimension "d102" = 6
  constraints: 14 end point, 14 point on circle, 7 centre point, 13 other
  measures "d102" distance between parallel lines of L3 L23
extrude "押し出し17" cut sketch "スケッチ10" against normal blind 4 contours A14 L25 A15 A16 A17 L28 A18 L23 A13
sketch "スケッチ11" plane through (0, 0, 0) normal (0, 0, 1) x (1, 0, 0)
  line L0 (95.9695, -37.3581) -> (66.885, -12.8501) projected
  arc A0 (66.885, -12.8501) -> (71.2186, -9.9571) centre (65.4443, -6) ccw projected
  arc A1 (71.2186, -9.9571) -> (74.0499, -9) centre (70.4443, -3) ccw projected
  line L1 (74.0499, -9) -> (80.2841, -9) projected
  arc A2 (80.2841, -9) -> (83.1155, -9.9571) centre (83.8897, -3) ccw projected
  arc A3 (83.1155, -9.9571) -> (92.3897, -12.0622) centre (88.8897, -6) ccw projected
  arc A4 (92.3897, -12.0622) -> (98.885, -12.3268) centre (95.8897, -6) ccw projected
  line L2 (98.885, -12.3268) -> (98.885, -29.6726) projected
  arc A5 (98.885, -29.6726) -> (95.9695, -37.3581) centre (111.885, -39) ccw projected
  line L3 (57.4443, -3) -> (54.4443, -3) projected
  arc A6 (52.4443, -3) -> (54.4443, -3) centre (53.4443, -3) ccw projected
  line L4 (52.4443, -3) -> (49.4443, -3) projected
  line L5 (49.4443, -3) -> (49.4443, -6) projected
  line L6 (49.4443, -6) -> (102.2194, -50.4706) projected
  arc A7 (102.2194, -50.4706) -> (121.0577, -50.8686) centre (111.885, -39) ccw projected
  line L7 (121.0577, -50.8686) -> (127.6513, -45.7727) projected
  line L8 (127.6513, -45.7727) -> (119.127, -45.896) projected
  arc A8 (104.885, -31.8586) -> (119.127, -45.896) centre (111.885, -39) ccw projected
  line L9 (104.885, -31.8586) -> (104.885, -3) projected
  line L10 (104.885, -3) -> (101.8897, -3) projected
  arc A9 (99.8897, -3) -> (101.8897, -3) centre (100.8897, -3) ccw projected
  line L11 (99.8897, -3) -> (96.8897, -3) projected
  line L12 (96.8897, -3) -> (96.8897, -6) projected
  arc A10 (94.8897, -6) -> (96.8897, -6) centre (95.8897, -6) ccw projected
  line L13 (94.8897, -6) -> (89.8897, -6) projected
  arc A11 (87.8897, -6) -> (89.8897, -6) centre (88.8897, -6) ccw projected
  line L14 (87.8897, -6) -> (87.8897, -3) projected
  line L15 (87.8897, -3) -> (84.8897, -3) projected
  arc A12 (82.8897, -3) -> (84.8897, -3) centre (83.8897, -3) ccw projected
  line L16 (82.8897, -3) -> (71.4443, -3) projected
  arc A13 (69.4443, -3) -> (71.4443, -3) centre (70.4443, -3) ccw projected
  line L17 (69.4443, -3) -> (66.4443, -3) projected
  line L18 (66.4443, -3) -> (66.4443, -6) projected
  arc A14 (64.4443, -6) -> (66.4443, -6) centre (65.4443, -6) ccw projected
  line L19 (64.4443, -6) -> (59.4443, -6) projected
  arc A15 (57.4443, -6) -> (59.4443, -6) centre (58.4443, -6) ccw projected
  line L20 (57.4443, -6) -> (57.4443, -3) projected
  point P0 (0, 0)
fillet "フィレット1" radius 1 9 edges at (98.885, -12.3268, -2) (92.3897, -12.0622, -2) (83.1155, -9.9571, -2) (80.2841, -9, -2) (98.885, -29.6726, -2) (74.0499, -9, -2) (71.2186, -9.9571, -2) (66.885, -12.8501, -2) (95.9695, -37.3581, -2)
sketch "スケッチ12" plane through (0, 0, 0) normal (0, 0, 1) x (1, 0, 0)
  line L0 (94.615, -36.2167) -> (68.2365, -13.989) projected
  arc A0 (68.4513, -12.3212) -> (68.2365, -13.989) centre (68.8809, -13.2243) ccw projected
  arc A1 (68.4513, -12.3212) -> (70.9856, -10.2772) centre (65.4443, -6) ccw projected
  arc A2 (71.6106, -9.9022) -> (70.9856, -10.2772) centre (71.7772, -10.8882) ccw projected
  arc A3 (71.6106, -9.9022) -> (73.8332, -9.125) centre (70.4443, -3) ccw projected
  arc A4 (74.3173, -9) -> (73.8332, -9.125) centre (74.3173, -10) ccw projected
  line L1 (74.3173, -9) -> (80.0167, -9) projected
  arc A5 (80.5008, -9.125) -> (80.0167, -9) centre (80.0167, -10) ccw projected
  arc A6 (80.5008, -9.125) -> (82.7234, -9.9022) centre (83.8897, -3) ccw projected
  arc A7 (83.3484, -10.2772) -> (82.7234, -9.9022) centre (82.5568, -10.8882) ccw projected
  arc A8 (83.3484, -10.2772) -> (91.9522, -12.2945) centre (88.8897, -6) ccw projected
  arc A9 (92.8272, -12.2945) -> (91.9522, -12.2945) centre (92.3897, -13.1937) ccw projected
  arc A10 (92.8272, -12.2945) -> (97.6356, -12.7788) centre (95.8897, -6) ccw projected
  arc A11 (98.885, -13.7472) -> (97.6356, -12.7788) centre (97.885, -13.7472) ccw projected
  line L2 (98.885, -13.7472) -> (98.885, -29.3564) projected
  arc A12 (98.7086, -29.9236) -> (98.885, -29.3564) centre (97.885, -29.3564) ccw projected
  arc A13 (98.7086, -29.9236) -> (96.2374, -35.6607) centre (111.885, -39) ccw projected
  arc A14 (94.615, -36.2167) -> (96.2374, -35.6607) centre (95.2594, -35.452) ccw projected
  line L3 (57.4443, -3) -> (54.4443, -3) projected
  arc A15 (52.4443, -3) -> (54.4443, -3) centre (53.4443, -3) ccw projected
  line L4 (52.4443, -3) -> (49.4443, -3) projected
  line L5 (49.4443, -3) -> (49.4443, -6) projected
  line L6 (49.4443, -6) -> (102.2194, -50.4706) projected
  arc A16 (102.2194, -50.4706) -> (121.0577, -50.8686) centre (111.885, -39) ccw projected
  line L7 (121.0577, -50.8686) -> (127.6513, -45.7727) projected
  line L8 (127.6513, -45.7727) -> (119.127, -45.896) projected
  arc A17 (104.885, -31.8586) -> (119.127, -45.896) centre (111.885, -39) ccw projected
  line L9 (104.885, -31.8586) -> (104.885, -3) projected
  line L10 (104.885, -3) -> (101.8897, -3) projected
  arc A18 (99.8897, -3) -> (101.8897, -3) centre (100.8897, -3) ccw projected
  line L11 (99.8897, -3) -> (96.8897, -3) projected
  line L12 (96.8897, -3) -> (96.8897, -6) projected
  arc A19 (94.8897, -6) -> (96.8897, -6) centre (95.8897, -6) ccw projected
  line L13 (94.8897, -6) -> (89.8897, -6) projected
  arc A20 (87.8897, -6) -> (89.8897, -6) centre (88.8897, -6) ccw projected
  line L14 (87.8897, -6) -> (87.8897, -3) projected
  line L15 (87.8897, -3) -> (84.8897, -3) projected
  arc A21 (82.8897, -3) -> (84.8897, -3) centre (83.8897, -3) ccw projected
  line L16 (82.8897, -3) -> (71.4443, -3) projected
  arc A22 (69.4443, -3) -> (71.4443, -3) centre (70.4443, -3) ccw projected
  line L17 (69.4443, -3) -> (66.4443, -3) projected
  line L18 (66.4443, -3) -> (66.4443, -6) projected
  arc A23 (64.4443, -6) -> (66.4443, -6) centre (65.4443, -6) ccw projected
  line L19 (64.4443, -6) -> (59.4443, -6) projected
  arc A24 (57.4443, -6) -> (59.4443, -6) centre (58.4443, -6) ccw projected
  line L20 (57.4443, -6) -> (57.4443, -3) projected
  line L21 (66.3034, -16.2831) -> (92.6819, -38.5108)
  arc A25 (92.6819, -38.5108) -> (99.1713, -36.2868) centre (95.2594, -35.452) ccw
  arc A26 (101.1792, -31.6254) -> (99.1713, -36.2868) centre (111.885, -39) ccw
  arc A27 (101.1792, -31.6254) -> (101.885, -29.3564) centre (97.885, -29.3564) ccw
  line L22 (101.885, -29.3564) -> (101.885, -13.7472)
  arc A28 (101.885, -13.7472) -> (96.8874, -9.8736) centre (97.885, -13.7472) ccw
  arc A29 (94.1397, -9.5969) -> (96.8874, -9.8736) centre (95.8897, -6) ccw
  arc A30 (94.1397, -9.5969) -> (90.6397, -9.5969) centre (92.3897, -13.1937) ccw
  arc A31 (85.7232, -8.4441) -> (90.6397, -9.5969) centre (88.8897, -6) ccw
  arc A32 (85.7232, -8.4441) -> (83.2232, -6.9441) centre (82.5568, -10.8882) ccw
  arc A33 (81.9532, -6.5) -> (83.2232, -6.9441) centre (83.8897, -3) ccw
  arc A34 (81.9532, -6.5) -> (80.0167, -6) centre (80.0167, -10) ccw
  line L23 (80.0167, -6) -> (74.3173, -6)
  arc A35 (74.3173, -6) -> (72.3808, -6.5) centre (74.3173, -10) ccw
  arc A36 (71.1108, -6.9441) -> (72.3808, -6.5) centre (70.4443, -3) ccw
  arc A37 (71.1108, -6.9441) -> (68.6108, -8.4441) centre (71.7772, -10.8882) ccw
  arc A38 (67.1626, -9.6121) -> (68.6108, -8.4441) centre (65.4443, -6) ccw
  arc A39 (67.1626, -9.6121) -> (66.3034, -16.2831) centre (68.8809, -13.2243) ccw
  line L24 (83.522, -30.7923) -> (103.193, -7.448) construction
  line L25 (84.6691, -31.7589) -> (104.3401, -8.4146)
  line L26 (102.046, -6.4814) -> (82.375, -29.8258)
  arc A40 (82.375, -29.8258) -> (84.6691, -31.7589) centre (83.522, -30.7923) ccw
  arc A41 (104.3401, -8.4146) -> (102.046, -6.4814) centre (103.193, -7.448) ccw
  point P0 (0, 0)
  point P1 (93.3575, -19.1202)
  point P2 (96.582, -12.9657)
  point P3 (84.3081, -27.5316)
  point P4 (86.6022, -29.4648)
  point P5 (98.885, -14.8883)
  dimension "d106" = 3
  dimension "d107" = 3
  constraints: 34 point on circle, 17 centre point, 14 end point, 4 tangent, 2 point on line, 1 midpoint, 1 parallel, 1 perpendicular, 17 other
  measures "d106" radial gap between concentric circles of A0 A39
  measures "d107" diameter of A41
extrude "押し出し18" add sketch "スケッチ12" against normal blind 5 contours L0 L26 A10 A11 L2 L25
fillet "フィレット2" radius 1 4 edges at (96.582, -12.9657, -2) (98.885, -14.8883, -2) (86.6022, -29.4648, -2) (84.3081, -27.5316, -2)
sketch "スケッチ13" plane through (0, 0, -2.55) normal (0, 0, 1) x (1, 0, 0)
  point P0 (0, 0)
sketch "スケッチ14" plane through (0, 0, 0) normal (0, 0, 1) x (1, 0, 0)
  circle A0 centre (111.885, -39) radius 3 projected
  line L0 (104.885, -3) -> (104.8897, -3) projected
  line L1 (104.885, -31.8586) -> (104.885, -3) projected
  arc A1 (104.885, -31.8586) -> (119.127, -45.896) centre (111.885, -39) ccw projected
  line L2 (127.6513, -45.7727) -> (119.127, -45.896) projected
  line L3 (126.8081, -37.4821) -> (127.6513, -45.7727) projected
  arc A2 (126.8081, -37.4821) -> (124.1514, -30.3665) centre (111.885, -39) ccw projected
  line L4 (104.8897, -3) -> (124.1514, -30.3665) projected
  circle A3 centre (111.885, -39) radius 8
  arc A4 (107.885, -33.2554) -> (117.6869, -42.9165) centre (111.885, -39) ccw
  line L5 (107.885, -33.2554) -> (107.885, -12.468)
  line L6 (107.885, -12.468) -> (121.6981, -32.0932)
  arc A5 (123.8235, -37.7857) -> (121.6981, -32.0932) centre (111.885, -39) ccw
  line L7 (123.8235, -37.7857) -> (124.3355, -42.8203)
  line L8 (124.3355, -42.8203) -> (117.6869, -42.9165)
  point P0 (0, 0)
  point P1 (107.885, -32.0718)
  point P2 (118.8704, -42.8994)
  dimension "d111" = 5
  dimension "d112" = 3
  constraints: 8 end point, 4 point on circle, 3 centre point, 5 other
  measures "d111" radial gap between concentric circles of A0 A3
  measures "d112" distance between parallel lines of L2 L8
extrude "押し出し19" cut sketch "スケッチ14" against normal blind 4 contours A3 L5 L6 A5 L7 L8
sketch "スケッチ15" plane through (0, 0, -2.55) normal (0, 0, 1) x (1, 0, 0)
  arc A0 (123.8235, -37.7857) -> (121.6981, -32.0932) centre (111.885, -39) ccw projected
  line L0 (123.8235, -37.7857) -> (124.3355, -42.8203) projected
  line L1 (124.3355, -42.8203) -> (118.8704, -42.8994) projected
  arc A1 (118.8704, -42.8994) -> (107.885, -32.0718) centre (111.885, -39) ccw projected
  line L2 (107.885, -32.0718) -> (107.885, -12.468) projected
  line L3 (107.885, -12.468) -> (121.6981, -32.0932) projected
  circle A2 centre (111.885, -39) radius 3 projected
  line L4 (104.885, -3) -> (104.8897, -3) projected
  line L5 (104.885, -31.8586) -> (104.885, -3) projected
  arc A3 (104.885, -31.8586) -> (119.127, -45.896) centre (111.885, -39) ccw projected
  line L6 (127.6513, -45.7727) -> (119.127, -45.896) projected
  line L7 (126.8081, -37.4821) -> (127.6513, -45.7727) projected
  arc A4 (126.8081, -37.4821) -> (124.1514, -30.3665) centre (111.885, -39) ccw projected
  line L8 (104.8897, -3) -> (124.1514, -30.3665) projected
  line L9 (111.885, -39) -> (128.504, -27.3029) construction
  line L10 (112.7484, -40.2266) -> (129.3674, -28.5295)
  line L11 (127.6407, -26.0763) -> (111.0217, -37.7734)
  arc A5 (111.0217, -37.7734) -> (112.7484, -40.2266) centre (111.885, -39) ccw
  arc A6 (129.3674, -28.5295) -> (127.6407, -26.0763) centre (128.504, -27.3029) ccw
  line L12 (107.885, -12.468) -> (121.6981, -32.0932) projected
  point P0 (0, 0)
  point P1 (120.1945, -33.1514)
  point P2 (120.8347, -30.8665)
  point P3 (117.4477, -33.2505)
  point P4 (119.1744, -35.7037)
  point P5 (122.4845, -33.374)
  dimension "d115" = 3
  constraints: 8 end point, 4 point on circle, 4 tangent, 2 centre point, 1 coincident, 1 midpoint, 1 parallel, 1 perpendicular
  measures "d115" diameter of A6
extrude "押し出し20" add sketch "スケッチ15" against normal blind 2.45 contours L10 A1 L11 L3 A0
fillet "フィレット3" radius 1 8 edges at (122.4845, -33.374, -3.275) (119.1744, -35.7037, -3.275) (117.4477, -33.2505, -3.275) (120.8347, -30.8665, -3.275) (107.885, -12.468, -3.275) (107.885, -32.0718, -3.275) (118.8704, -42.8994, -3.275) (124.3355, -42.8203, -3.275)
sketch "スケッチ16" plane through (0, 0, -2.55) normal (0, 0, 1) x (1, 0, 0)
  arc A0 (123.8235, -37.7857) -> (123.011, -34.5042) centre (111.885, -39) ccw projected
  line L0 (123.8235, -37.7857) -> (124.2252, -41.735) projected
  arc A1 (123.2447, -42.8361) -> (124.2252, -41.735) centre (123.2303, -41.8362) ccw projected
  line L1 (123.2447, -42.8361) -> (120.4273, -42.8769) projected
  arc A2 (119.4653, -41.5573) -> (120.4273, -42.8769) centre (120.4128, -41.877) ccw projected
  arc A3 (119.4653, -41.5573) -> (119.4487, -36.3939) centre (111.885, -39) ccw projected
  arc A4 (119.8185, -35.2504) -> (119.4487, -36.3939) centre (120.3941, -36.0681) ccw projected
  line L2 (119.8185, -35.2504) -> (121.5083, -34.0611) projected
  arc A5 (123.011, -34.5042) -> (121.5083, -34.0611) centre (122.0839, -34.8788) ccw projected
  line L3 (120.017, -31.4421) -> (118.0918, -32.7971) projected
  arc A6 (116.8906, -32.7594) -> (118.0918, -32.7971) centre (117.5163, -31.9794) ccw projected
  arc A7 (116.8906, -32.7594) -> (109.2184, -31.4575) centre (111.885, -39) ccw projected
  arc A8 (107.885, -30.5147) -> (109.2184, -31.4575) centre (108.885, -30.5147) ccw projected
  line L4 (107.885, -30.5147) -> (107.885, -15.6261) projected
  arc A9 (109.7028, -15.0506) -> (107.885, -15.6261) centre (108.885, -15.6261) ccw projected
  line L5 (109.7028, -15.0506) -> (120.2592, -30.0488) projected
  arc A10 (120.017, -31.4421) -> (120.2592, -30.0488) centre (119.4414, -30.6244) ccw projected
  circle A11 centre (111.885, -39) radius 3 projected
  line L6 (104.885, -3) -> (104.8897, -3) projected
  line L7 (104.885, -31.8586) -> (104.885, -3) projected
  arc A12 (104.885, -31.8586) -> (119.127, -45.896) centre (111.885, -39) ccw projected
  line L8 (127.6513, -45.7727) -> (119.127, -45.896) projected
  line L9 (126.8081, -37.4821) -> (127.6513, -45.7727) projected
  arc A13 (126.8081, -37.4821) -> (124.1514, -30.3665) centre (111.885, -39) ccw projected
  line L10 (104.8897, -3) -> (124.1514, -30.3665) projected
  line L11 (124.8759, -15.5852) -> (100.2505, -32.9176) construction
  line L12 (124.0126, -14.3586) -> (99.3871, -31.691)
  line L13 (101.1138, -34.1442) -> (125.7393, -16.8118)
  arc A14 (125.7393, -16.8118) -> (124.0126, -14.3586) centre (124.8759, -15.5852) ccw
  arc A15 (99.3871, -31.691) -> (101.1138, -34.1442) centre (100.2505, -32.9176) ccw
  point P0 (0, 0)
  point P1 (112.5632, -24.2514)
  point P2 (114.981, -22.5497)
  point P3 (107.885, -29.3784)
  point P4 (115.8443, -23.7763)
  point P5 (114.1176, -21.3231)
  point P6 (107.885, -25.7098)
  dimension "d119" = 3
  constraints: 8 end point, 4 point on circle, 4 tangent, 2 centre point, 2 midpoint, 1 parallel, 1 perpendicular, 1 point on line
  measures "d119" diameter of A15
extrude "押し出し21" add sketch "スケッチ16" against normal blind 2.45 contours L13 L4 L12 L5
fillet "フィレット4" radius 1 4 edges at (114.1176, -21.3231, -3.275) (115.8443, -23.7763, -3.275) (107.885, -29.3784, -3.275) (107.885, -25.7098, -3.275)
sketch "スケッチ17" plane through (0, 0, -5) normal (0, 0, -1) x (-1, 0, 0)
  line L0 (-98.885, -17.6269) -> (-98.885, -29.3564) projected
  arc A0 (-98.885, -29.3564) -> (-98.7086, -29.9236) centre (-97.885, -29.3564) ccw projected
  arc A1 (-96.2374, -35.6607) -> (-98.7086, -29.9236) centre (-111.885, -39) ccw projected
  arc A2 (-96.2374, -35.6607) -> (-94.615, -36.2167) centre (-95.2594, -35.452) ccw projected
  line L1 (-94.615, -36.2167) -> (-87.3669, -30.1091) projected
  arc A3 (-87.3669, -30.1091) -> (-87.2466, -28.7001) centre (-88.0113, -29.3444) ccw projected
  line L2 (-87.2466, -28.7001) -> (-97.1203, -16.9825) projected
  arc A4 (-97.1203, -16.9825) -> (-98.885, -17.6269) centre (-97.885, -17.6269) ccw projected
  line L3 (-95.2693, -14.5236) -> (-84.9525, -26.7669) projected
  arc A5 (-84.9525, -26.7669) -> (-83.5434, -26.8873) centre (-84.1878, -26.1225) ccw projected
  line L4 (-83.5434, -26.8873) -> (-68.2365, -13.989) projected
  arc A6 (-68.2365, -13.989) -> (-68.4513, -12.3212) centre (-68.8809, -13.2243) ccw projected
  arc A7 (-70.9856, -10.2772) -> (-68.4513, -12.3212) centre (-65.4443, -6) ccw projected
  arc A8 (-70.9856, -10.2772) -> (-71.6106, -9.9022) centre (-71.7772, -10.8882) ccw projected
  arc A9 (-73.8332, -9.125) -> (-71.6106, -9.9022) centre (-70.4443, -3) ccw projected
  arc A10 (-73.8332, -9.125) -> (-74.3173, -9) centre (-74.3173, -10) ccw projected
  line L5 (-74.3173, -9) -> (-80.0167, -9) projected
  arc A11 (-80.0167, -9) -> (-80.5008, -9.125) centre (-80.0167, -10) ccw projected
  arc A12 (-82.7234, -9.9022) -> (-80.5008, -9.125) centre (-83.8897, -3) ccw projected
  arc A13 (-82.7234, -9.9022) -> (-83.3484, -10.2772) centre (-82.5568, -10.8882) ccw projected
  arc A14 (-91.9522, -12.2945) -> (-83.3484, -10.2772) centre (-88.8897, -6) ccw projected
  arc A15 (-91.9522, -12.2945) -> (-92.8272, -12.2945) centre (-92.3897, -13.1937) ccw projected
  arc A16 (-94.6777, -12.8943) -> (-92.8272, -12.2945) centre (-95.8897, -6) ccw projected
  arc A17 (-94.6777, -12.8943) -> (-95.2693, -14.5236) centre (-94.5046, -13.8792) ccw projected
  line L6 (-57.4443, -3) -> (-54.4443, -3) projected
  arc A18 (-54.4443, -3) -> (-52.4443, -3) centre (-53.4443, -3) ccw projected
  line L7 (-52.4443, -3) -> (-49.4443, -3) projected
  line L8 (-49.4443, -3) -> (-49.4443, -6) projected
  line L9 (-49.4443, -6) -> (-102.2194, -50.4706) projected
  arc A19 (-121.0577, -50.8686) -> (-102.2194, -50.4706) centre (-111.885, -39) ccw projected
  line L10 (-121.0577, -50.8686) -> (-127.6513, -45.7727) projected
  line L11 (-127.6513, -45.7727) -> (-119.127, -45.896) projected
  arc A20 (-119.127, -45.896) -> (-104.885, -31.8586) centre (-111.885, -39) ccw projected
  line L12 (-104.885, -31.8586) -> (-104.885, -3) projected
  line L13 (-104.885, -3) -> (-101.8897, -3) projected
  arc A21 (-101.8897, -3) -> (-99.8897, -3) centre (-100.8897, -3) ccw projected
  line L14 (-99.8897, -3) -> (-96.8897, -3) projected
  line L15 (-96.8897, -3) -> (-96.8897, -6) projected
  arc A22 (-96.8897, -6) -> (-94.8897, -6) centre (-95.8897, -6) ccw projected
  line L16 (-94.8897, -6) -> (-89.8897, -6) projected
  arc A23 (-89.8897, -6) -> (-87.8897, -6) centre (-88.8897, -6) ccw projected
  line L17 (-87.8897, -6) -> (-87.8897, -3) projected
  line L18 (-87.8897, -3) -> (-84.8897, -3) projected
  arc A24 (-84.8897, -3) -> (-82.8897, -3) centre (-83.8897, -3) ccw projected
  line L19 (-82.8897, -3) -> (-71.4443, -3) projected
  arc A25 (-71.4443, -3) -> (-69.4443, -3) centre (-70.4443, -3) ccw projected
  line L20 (-69.4443, -3) -> (-66.4443, -3) projected
  line L21 (-66.4443, -3) -> (-66.4443, -6) projected
  arc A26 (-66.4443, -6) -> (-64.4443, -6) centre (-65.4443, -6) ccw projected
  line L22 (-64.4443, -6) -> (-59.4443, -6) projected
  arc A27 (-59.4443, -6) -> (-57.4443, -6) centre (-58.4443, -6) ccw projected
  line L23 (-57.4443, -6) -> (-57.4443, -3) projected
  line L24 (-107.885, -23.7831) -> (-107.885, -15.6261) projected
  arc A28 (-107.885, -15.6261) -> (-109.7028, -15.0506) centre (-108.885, -15.6261) ccw projected
  line L25 (-109.7028, -15.0506) -> (-113.5421, -20.5053) projected
  arc A29 (-113.5421, -20.5053) -> (-113.2999, -21.8986) centre (-112.7243, -21.0809) ccw projected
  line L26 (-113.2999, -21.8986) -> (-109.4606, -24.6009) projected
  arc A30 (-109.4606, -24.6009) -> (-107.885, -23.7831) centre (-108.885, -23.7831) ccw projected
  arc A31 (-123.011, -34.5042) -> (-123.8235, -37.7857) centre (-111.885, -39) ccw projected
  line L27 (-123.8235, -37.7857) -> (-124.2252, -41.735) projected
  arc A32 (-124.2252, -41.735) -> (-123.2447, -42.8361) centre (-123.2303, -41.8362) ccw projected
  line L28 (-123.2447, -42.8361) -> (-120.4273, -42.8769) projected
  arc A33 (-120.4273, -42.8769) -> (-119.4653, -41.5573) centre (-120.4128, -41.877) ccw projected
  arc A34 (-119.4487, -36.3939) -> (-119.4653, -41.5573) centre (-111.885, -39) ccw projected
  arc A35 (-119.4487, -36.3939) -> (-119.8185, -35.2504) centre (-120.3941, -36.0681) ccw projected
  line L29 (-119.8185, -35.2504) -> (-121.5083, -34.0611) projected
  arc A36 (-121.5083, -34.0611) -> (-123.011, -34.5042) centre (-122.0839, -34.8788) ccw projected
  line L30 (-108.3095, -29.0797) -> (-115.0266, -24.3519) projected
  arc A37 (-115.0266, -24.3519) -> (-116.4199, -24.5941) centre (-115.6022, -25.1696) ccw projected
  line L31 (-116.4199, -24.5941) -> (-120.2592, -30.0488) projected
  arc A38 (-120.2592, -30.0488) -> (-120.017, -31.4421) centre (-119.4414, -30.6244) ccw projected
  line L32 (-120.017, -31.4421) -> (-118.0918, -32.7971) projected
  arc A39 (-118.0918, -32.7971) -> (-116.8906, -32.7594) centre (-117.5163, -31.9794) ccw projected
  arc A40 (-109.2184, -31.4575) -> (-116.8906, -32.7594) centre (-111.885, -39) ccw projected
  arc A41 (-109.2184, -31.4575) -> (-107.885, -30.5147) centre (-108.885, -30.5147) ccw projected
  line L33 (-107.885, -30.5147) -> (-107.885, -29.8974) projected
  arc A42 (-107.885, -29.8974) -> (-108.3095, -29.0797) centre (-108.885, -29.8974) ccw projected
  circle A43 centre (-111.885, -39) radius 3 projected
  line L34 (-104.885, -3) -> (-104.8897, -3) projected
  line L35 (-104.885, -31.8586) -> (-104.885, -3) projected
  arc A44 (-119.127, -45.896) -> (-104.885, -31.8586) centre (-111.885, -39) ccw projected
  line L36 (-127.6513, -45.7727) -> (-119.127, -45.896) projected
  line L37 (-126.8081, -37.4821) -> (-127.6513, -45.7727) projected
  arc A45 (-124.1514, -30.3665) -> (-126.8081, -37.4821) centre (-111.885, -39) ccw projected
  line L38 (-104.8897, -3) -> (-124.1514, -30.3665) projected
  point P0 (0, 0)